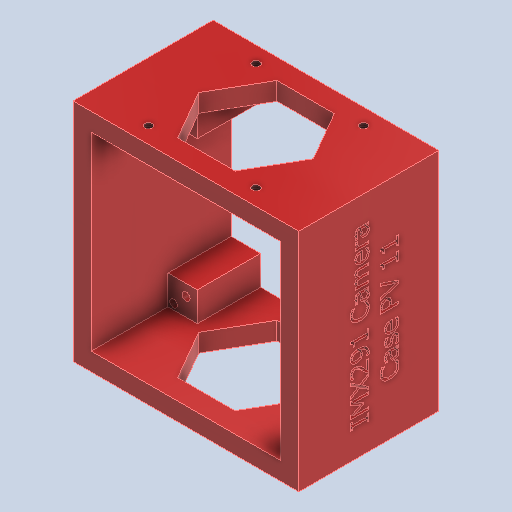
# Autodesk Inventor part: IMX291 Camera Case Base
Saved by Autodesk Inventor 2023 (Build 270158030, 158C)
## iProperties
Created: 2021-07-23
Part Number: IMX291 Camera Case Base
Material: PET Plastic
Document SubType Name: Modeling
Designer: robst
Density: 1.541 g/cm^3
Appearance: Red
Author: robst
Autodesk Inventor part; units mm, degrees
note: some values were not read from the file. Chosen so that the rebuilt part matches the saved one: direction of "Emboss2"; direction of "Hole3".
ref_plane "YZ Plane" through (0, 0, 0) normal (1, 0, 0) x (0, 1, 0)
ref_plane "XZ Plane" through (0, 0, 0) normal (0, 1, 0) x (-1, 0, 0)
ref_plane "XY Plane" through (0, 0, 0) normal (0, 0, 1) x (1, 0, 0)
sketch "Sketch8" plane through (0, 0, 0) normal (0, 0, 1) x (1, 0, 0)
  line L0 (-17, -17) -> (17, -17) construction
  line L1 (17, -17) -> (17, 17) construction
  line L2 (17, 17) -> (-17, 17) construction
  line L3 (-17, 17) -> (-17, -17) construction
  line L4 (-17, -17) -> (17, 17) construction
  line L5 (17, -17) -> (-17, 17) construction
  circle A0 centre (-17, 17) radius 0.9
  circle A1 centre (17, 17) radius 0.9
  circle A2 centre (17, -17) radius 0.9
  circle A3 centre (-17, -17) radius 0.9
  line L6 (-21, -21) -> (21, -21)
  line L7 (21, -21) -> (21, 21)
  line L8 (21, 21) -> (-21, 21)
  line L9 (-21, 21) -> (-21, -21)
  line L10 (-21, -21) -> (21, 21) construction
  line L11 (21, -21) -> (-21, 21) construction
  line L12 (-25, -25) -> (25, -25)
  line L13 (25, -25) -> (25, 25)
  line L14 (25, 25) -> (-25, 25)
  line L15 (-25, 25) -> (-25, -25)
  line L16 (-25, -25) -> (25, 25) construction
  line L17 (25, -25) -> (-25, 25) construction
  line L18 (0, 0) -> (9.8286, 0)
  line L19 (-14.5, -14.5) -> (14.5, -14.5) construction
  line L20 (14.5, -14.5) -> (14.5, 14.5) construction
  line L21 (14.5, 14.5) -> (-14.5, 14.5) construction
  line L22 (-14.5, 14.5) -> (-14.5, -14.5) construction
  line L23 (-14.5, -14.5) -> (14.5, 14.5) construction
  line L24 (14.5, -14.5) -> (-14.5, 14.5) construction
  line L25 (-21, 21) -> (-14.5, 21)
  line L26 (-14.5, 21) -> (-14.5, 14.5)
  line L27 (-14.5, 14.5) -> (-21, 14.5)
  line L28 (-21, 14.5) -> (-21, 21)
  line L29 (21, 21) -> (14.5, 21)
  line L30 (14.5, 21) -> (14.5, 14.5)
  line L31 (14.5, 14.5) -> (21, 14.5)
  line L32 (21, 14.5) -> (21, 21)
  line L33 (21, -21) -> (14.5, -21)
  line L34 (14.5, -21) -> (14.5, -14.5)
  line L35 (14.5, -14.5) -> (21, -14.5)
  line L36 (21, -14.5) -> (21, -21)
  line L37 (-21, -21) -> (-14.5, -21)
  line L38 (-14.5, -21) -> (-14.5, -14.5)
  line L39 (-14.5, -14.5) -> (-21, -14.5)
  line L40 (-21, -14.5) -> (-21, -21)
  point P0 (-25, 0)
  point P1 (-14.5, -21)
  dimension "d46" = 34
  dimension "d47" = 34
  dimension "d48" = 1.8
  dimension "d49" = 42
  dimension "d50" = 42
  dimension "d51" = 4
  dimension "d52" = 4
  dimension "d53" = 29
  dimension "d54" = 29
  dimension "d61" = 50
  dimension "d62" = 50
  constraints: 82 end point, 16 parallel, 9 midpoint, 8 horizontal, 8 perpendicular, 4 centre point, 4 coincident, 3 equal radius, 2 point on line
  measures "d46" distance of L0.start L0.end
  measures "d47" distance of L2.end L0.start
  measures "d48" diameter of A0
  measures "d49" distance of L7.end L8.end
  measures "d50" distance of L6.end L7.end
  measures "d51" distance between parallel lines of L8 L14
  measures "d52" distance from line of point (-25, 0) L9
  measures "d53" distance of L19.start L19.end
  measures "d54" distance of L20.end L19.end
  measures "d61" distance between parallel lines of L14 L12
  measures "d62" distance between parallel lines of L15 L13
extrude "Extrusion9" add sketch "Sketch8" against normal blind 14 contours L9 L39 L38 L6 | L34 L35 L7 L6 | L9 L8 L26 L27 | L31 L30 L8 L7 | L15 L14 L13 L12
sketch "Sketch9" plane through (0, 0, 0) normal (0, 0, 1) x (1, 0, 0)
  line L0 (21, 14.5) -> (21, -14.5) projected
  line L1 (-14.5, 21) -> (14.5, 21) projected
  line L2 (-21, -14.5) -> (-21, 14.5) projected
  line L3 (14.5, -21) -> (-14.5, -21) projected
  line L4 (-25, -25) -> (25, -25) projected
  line L5 (25, -25) -> (25, 25) projected
  line L6 (25, 25) -> (-25, 25) projected
  line L7 (-25, 25) -> (-25, -25) projected
  line L8 (-21, -21) -> (21, -21)
  line L9 (21, -21) -> (21, 21)
  line L10 (21, 21) -> (-21, 21)
  line L11 (-21, 21) -> (-21, -21)
  line L12 (-21, -21) -> (21, 21) construction
  line L13 (21, -21) -> (-21, 21) construction
  line L14 (-23, -23) -> (23, -23)
  line L15 (23, -23) -> (23, 23)
  line L16 (23, 23) -> (-23, 23)
  line L17 (-23, 23) -> (-23, -23)
  line L18 (-23, -23) -> (23, 23) construction
  line L19 (23, -23) -> (-23, 23) construction
  point P0 (0, 0)
  point P1 (-14.5, -21)
  constraints: 24 end point, 4 midpoint, 4 parallel, 2 perpendicular
extrude "Extrusion10" add sketch "Sketch9" along normal blind 17 contours L7 L6 L5 L4 | L17 L16 L15 L14
sketch "Sketch10" plane through (25, -25, -14) normal (1, 0, 0) x (0, 0, -1)
  line L0 (-31, 0) -> (0, 0) construction
  line L1 (-15.5, 0) -> (-15.5, 50) construction
  line L2 (0, 50) -> (-31, 50) construction
  line L3 (-15.5, 7.4068) -> (-15.5, 5.8574)
  line L4 (-15.5, 5.8574) -> (-15.9084, 5.8574)
  line L5 (-15.9084, 5.8574) -> (-15.9084, 6.3663)
  line L6 (-15.9084, 6.3663) -> (-19.0916, 6.3663)
  line L7 (-19.0916, 6.3663) -> (-19.0916, 5.8574)
  line L8 (-19.0916, 5.8574) -> (-19.5, 5.8574)
  line L9 (-19.5, 5.8574) -> (-19.5, 7.4068)
  line L10 (-19.5, 7.4068) -> (-19.0916, 7.4068)
  line L11 (-19.0916, 7.4068) -> (-19.0916, 6.8979)
  line L12 (-19.0916, 6.8979) -> (-15.9084, 6.8979)
  line L13 (-15.9084, 6.8979) -> (-15.9084, 7.4068)
  line L14 (-15.9084, 7.4068) -> (-15.5, 7.4068)
  line L15 (-15.5, 11.4943) -> (-15.5, 10.9627)
  line L16 (-15.5, 10.9627) -> (-18.9457, 10.9627)
  line L17 (-18.9457, 10.9627) -> (-16.6021, 9.919)
  line L18 (-16.6021, 9.919) -> (-16.6021, 9.5948)
  line L19 (-16.6021, 9.5948) -> (-18.9457, 8.5608)
  line L20 (-18.9457, 8.5608) -> (-15.5, 8.5608)
  line L21 (-15.5, 8.5608) -> (-15.5, 8.0648)
  line L22 (-15.5, 8.0648) -> (-19.5, 8.0648)
  line L23 (-19.5, 8.0648) -> (-19.5, 8.7909)
  line L24 (-19.5, 8.7909) -> (-17.2731, 9.7893)
  line L25 (-17.2731, 9.7893) -> (-19.5, 10.7553)
  line L26 (-19.5, 10.7553) -> (-19.5, 11.4943)
  line L27 (-19.5, 11.4943) -> (-15.5, 11.4943)
  line L28 (-15.5, 15.0697) -> (-15.5, 14.4603)
  line L29 (-15.5, 14.4603) -> (-17.0948, 13.4878)
  line L30 (-17.0948, 13.4878) -> (-15.5, 12.4959)
  line L31 (-15.5, 12.4959) -> (-15.5, 11.9222)
  line L32 (-15.5, 11.9222) -> (-17.5032, 13.1961)
  line L33 (-17.5032, 13.1961) -> (-19.5, 11.9611)
  line L34 (-19.5, 11.9611) -> (-19.5, 12.5705)
  line L35 (-19.5, 12.5705) -> (-17.9344, 13.5235)
  line L36 (-17.9344, 13.5235) -> (-19.5, 14.4959)
  line L37 (-19.5, 14.4959) -> (-19.5, 15.0697)
  line L38 (-19.5, 15.0697) -> (-17.5292, 13.8185)
  line L39 (-17.5292, 13.8185) -> (-15.5, 15.0697)
  line L40 (-15.5, 17.8509) -> (-15.5, 15.3841)
  line L41 (-15.5, 15.3841) -> (-16.0673, 15.3841)
  spline S0 degree 2 poles (-16.0673, 15.3841) (-16.3169, 15.6499) (-16.7804, 16.1232) (-17.03, 16.3501) knots 0 0 0 1 2 2 2
  spline S1 degree 2 poles (-17.03, 16.3501) (-17.5324, 16.8071) (-18.1353, 17.141) (-18.4562, 17.141) knots 0 0 0 1 2 2 2
  spline S2 degree 2 poles (-18.4562, 17.141) (-18.6248, 17.141) (-18.8776, 17.0373) (-18.9587, 16.9433) knots 0 0 0 1 2 2 2
  spline S3 degree 2 poles (-18.9587, 16.9433) (-19.0397, 16.8493) (-19.1207, 16.6029) (-19.1207, 16.4538) knots 0 0 0 1 2 2 2
  spline S4 degree 2 poles (-19.1207, 16.4538) (-19.1207, 16.3112) (-19.0494, 16.0194) (-18.9943, 15.8865) knots 0 0 0 1 2 2 2
  spline S5 degree 2 poles (-18.9943, 15.8865) (-18.9489, 15.7731) (-18.8193, 15.5624) (-18.7739, 15.4976) knots 0 0 0 1 2 2 2
  line L42 (-18.7739, 15.4976) -> (-18.7739, 15.4684)
  line L43 (-18.7739, 15.4684) -> (-19.3444, 15.4684)
  spline S6 degree 2 poles (-19.3444, 15.4684) (-19.4254, 15.6337) (-19.5843, 16.2269) (-19.5843, 16.4927) knots 0 0 0 1 2 2 2
  spline S7 degree 2 poles (-19.5843, 16.4927) (-19.5843, 17.0535) (-18.9911, 17.6856) (-18.4854, 17.6856) knots 0 0 0 1 2 2 2
  spline S8 degree 2 poles (-18.4854, 17.6856) (-18.2488, 17.6856) (-17.8533, 17.5754) (-17.6848, 17.4781) knots 0 0 0 1 2 2 2
  spline S9 degree 2 poles (-17.6848, 17.4781) (-17.5097, 17.3809) (-17.1661, 17.0989) (-17.0008, 16.9433) knots 0 0 0 1 2 2 2
  spline S10 degree 2 poles (-17.0008, 16.9433) (-16.7253, 16.6904) (-16.1353, 16.0713) (-15.9635, 15.8865) knots 0 0 0 1 2 2 2
  line L44 (-15.9635, 15.8865) -> (-15.9635, 17.8509)
  line L45 (-15.9635, 17.8509) -> (-15.5, 17.8509)
  spline S11 degree 2 poles (-18.2002, 18.2755) (-18.5081, 18.2755) (-19.0203, 18.4765) (-19.205, 18.6515) knots 0 0 0 1 2 2 2
  spline S12 degree 2 poles (-19.205, 18.6515) (-19.3833, 18.8169) (-19.581, 19.2998) (-19.581, 19.5462) knots 0 0 0 1 2 2 2
  spline S13 degree 2 poles (-19.581, 19.5462) (-19.581, 19.8217) (-19.3963, 20.269) (-19.2212, 20.4344) knots 0 0 0 1 2 2 2
  spline S14 degree 2 poles (-19.2212, 20.4344) (-19.0008, 20.6418) (-18.2877, 20.8687) (-17.7399, 20.8687) knots 0 0 0 1 2 2 2
  spline S15 degree 2 poles (-17.7399, 20.8687) (-17.2439, 20.8687) (-16.3558, 20.6451) (-16.0608, 20.4279) knots 0 0 0 1 2 2 2
  spline S16 degree 2 poles (-16.0608, 20.4279) (-15.7496, 20.1977) (-15.4222, 19.5494) (-15.4222, 19.0762) knots 0 0 0 1 2 2 2
  spline S17 degree 2 poles (-15.4222, 19.0762) (-15.4222, 18.9692) (-15.4449, 18.7261) (-15.4773, 18.6224) knots 0 0 0 1 2 2 2
  line L46 (-15.4773, 18.6224) -> (-15.9927, 18.6224)
  line L47 (-15.9927, 18.6224) -> (-15.9927, 18.6483)
  spline S18 degree 2 poles (-15.9927, 18.6483) (-15.9538, 18.7164) (-15.8857, 19.0016) (-15.8857, 19.1475) knots 0 0 0 1 2 2 2
  spline S19 degree 2 poles (-15.8857, 19.1475) (-15.8857, 19.6726) (-16.5794, 20.2723) (-17.2212, 20.3144) knots 0 0 0 1 2 2 2
  spline S20 degree 2 poles (-17.2212, 20.3144) (-17.0754, 20.1005) (-16.9425, 19.7115) (-16.9425, 19.4814) knots 0 0 0 1 2 2 2
  spline S21 degree 2 poles (-16.9425, 19.4814) (-16.9425, 19.2609) (-17.0397, 18.8947) (-17.1791, 18.7099) knots 0 0 0 1 2 2 2
  spline S22 degree 2 poles (-17.1791, 18.7099) (-17.3444, 18.4959) (-17.8468, 18.2755) (-18.2002, 18.2755) knots 0 0 0 1 2 2 2
  spline S23 degree 2 poles (-17.8598, 20.3274) (-18.265, 20.3274) (-18.7771, 20.1783) (-18.9165, 20.0454) knots 0 0 0 1 2 2 2
  spline S24 degree 2 poles (-18.9165, 20.0454) (-19.0462, 19.9287) (-19.1434, 19.6856) (-19.1434, 19.5429) knots 0 0 0 1 2 2 2
  spline S25 degree 2 poles (-19.1434, 19.5429) (-19.1434, 19.2123) (-18.6702, 18.8201) (-18.2229, 18.8201) knots 0 0 0 1 2 2 2
  spline S26 degree 2 poles (-18.2229, 18.8201) (-17.97, 18.8201) (-17.6426, 18.9498) (-17.5259, 19.0924) knots 0 0 0 1 2 2 2
  spline S27 degree 2 poles (-17.5259, 19.0924) (-17.4417, 19.1961) (-17.3865, 19.4522) (-17.3865, 19.6013) knots 0 0 0 1 2 2 2
  spline S28 degree 2 poles (-17.3865, 19.6013) (-17.3865, 19.7731) (-17.5065, 20.1686) (-17.607, 20.3177) knots 0 0 0 1 2 2 2
  spline S29 degree 2 poles (-17.607, 20.3177) (-17.6459, 20.3209) (-17.7788, 20.3274) (-17.8598, 20.3274) knots 0 0 0 1 2 2 2
  line L48 (-15.5, 23.6532) -> (-15.5, 21.7018)
  line L49 (-15.5, 21.7018) -> (-15.9084, 21.7018)
  line L50 (-15.9084, 21.7018) -> (-15.9084, 22.4279)
  line L51 (-15.9084, 22.4279) -> (-18.5891, 22.4279)
  line L52 (-18.5891, 22.4279) -> (-18.5891, 21.7018)
  line L53 (-18.5891, 21.7018) -> (-18.9554, 21.7018)
  spline S30 degree 2 poles (-18.9554, 21.7018) (-18.9554, 22.1135) (-19.1888, 22.5024) (-19.513, 22.5284) knots 0 0 0 1 2 2 2
  line L54 (-19.513, 22.5284) -> (-19.513, 22.9433)
  line L55 (-19.513, 22.9433) -> (-15.9084, 22.9433)
  line L56 (-15.9084, 22.9433) -> (-15.9084, 23.6532)
  line L57 (-15.9084, 23.6532) -> (-15.5, 23.6532)
  spline S31 degree 2 poles (-15.4287, 27.7828) (-15.4287, 27.3938) (-15.6912, 26.7358) (-15.9538, 26.4959) knots 0 0 0 1 2 2 2
  spline S32 degree 2 poles (-15.9538, 26.4959) (-16.2131, 26.2561) (-16.9911, 25.9935) (-17.4968, 25.9935) knots 0 0 0 1 2 2 2
  spline S33 degree 2 poles (-17.4968, 25.9935) (-17.9992, 25.9935) (-18.7447, 26.2496) (-19.0203, 26.4927) knots 0 0 0 1 2 2 2
  spline S34 degree 2 poles (-19.0203, 26.4927) (-19.2893, 26.7326) (-19.5713, 27.3874) (-19.5713, 27.7925) knots 0 0 0 1 2 2 2
  spline S35 degree 2 poles (-19.5713, 27.7925) (-19.5713, 27.9935) (-19.513, 28.3468) (-19.4676, 28.4959) knots 0 0 0 1 2 2 2
  spline S36 degree 2 poles (-19.4676, 28.4959) (-19.4254, 28.6256) (-19.3055, 28.8947) (-19.2342, 29.0276) knots 0 0 0 1 2 2 2
  line L58 (-19.2342, 29.0276) -> (-18.5924, 29.0276)
  line L59 (-18.5924, 29.0276) -> (-18.5924, 28.9854)
  spline S37 degree 2 poles (-18.5924, 28.9854) (-18.6572, 28.9141) (-18.8387, 28.6937) (-18.9263, 28.5348) knots 0 0 0 1 2 2 2
  spline S38 degree 2 poles (-18.9263, 28.5348) (-19.0105, 28.3825) (-19.1175, 28.0227) (-19.1175, 27.7893) knots 0 0 0 1 2 2 2
  spline S39 degree 2 poles (-19.1175, 27.7893) (-19.1175, 27.5332) (-18.9068, 27.0762) (-18.7058, 26.9044) knots 0 0 0 1 2 2 2
  spline S40 degree 2 poles (-18.7058, 26.9044) (-18.5016, 26.7358) (-17.8825, 26.5478) (-17.4968, 26.5478) knots 0 0 0 1 2 2 2
  spline S41 degree 2 poles (-17.4968, 26.5478) (-17.0851, 26.5478) (-16.4919, 26.7455) (-16.2877, 26.9173) knots 0 0 0 1 2 2 2
  spline S42 degree 2 poles (-16.2877, 26.9173) (-16.09, 27.0859) (-15.889, 27.5365) (-15.889, 27.7893) knots 0 0 0 1 2 2 2
  spline S43 degree 2 poles (-15.889, 27.7893) (-15.889, 28.0194) (-16.0024, 28.4117) (-16.0867, 28.564) knots 0 0 0 1 2 2 2
  spline S44 degree 2 poles (-16.0867, 28.564) (-16.171, 28.7099) (-16.346, 28.9271) (-16.4076, 28.9887) knots 0 0 0 1 2 2 2
  line L60 (-16.4076, 28.9887) -> (-16.4076, 29.0276)
  line L61 (-16.4076, 29.0276) -> (-15.7723, 29.0276)
  spline S45 degree 2 poles (-15.7723, 29.0276) (-15.7107, 28.8947) (-15.5972, 28.6613) (-15.5454, 28.4959) knots 0 0 0 1 2 2 2
  spline S46 degree 2 poles (-15.5454, 28.4959) (-15.487, 28.3209) (-15.4287, 28.0227) (-15.4287, 27.7828) knots 0 0 0 1 2 2 2
  spline S47 degree 2 poles (-15.8177, 31.1572) (-15.7723, 31.0956) (-15.6102, 30.8882) (-15.5616, 30.7909) knots 0 0 0 1 2 2 2
  spline S48 degree 2 poles (-15.5616, 30.7909) (-15.4903, 30.658) (-15.4157, 30.4084) (-15.4157, 30.1815) knots 0 0 0 1 2 2 2
  spline S49 degree 2 poles (-15.4157, 30.1815) (-15.4157, 29.9968) (-15.5551, 29.6629) (-15.6815, 29.5365) knots 0 0 0 1 2 2 2
  spline S50 degree 2 poles (-15.6815, 29.5365) (-15.8047, 29.4165) (-16.1677, 29.2707) (-16.3687, 29.2707) knots 0 0 0 1 2 2 2
  spline S51 degree 2 poles (-16.3687, 29.2707) (-16.6799, 29.2707) (-17.1207, 29.5332) (-17.2472, 29.8185) knots 0 0 0 1 2 2 2
  spline S52 degree 2 poles (-17.2472, 29.8185) (-17.3639, 30.0713) (-17.4514, 30.7585) (-17.4741, 31.1572) knots 0 0 0 1 2 2 2
  line L62 (-17.4741, 31.1572) -> (-17.5713, 31.1572)
  spline S53 degree 2 poles (-17.5713, 31.1572) (-17.7464, 31.1572) (-17.9635, 31.0502) (-18.0251, 30.953) knots 0 0 0 1 2 2 2
  spline S54 degree 2 poles (-18.0251, 30.953) (-18.0867, 30.8558) (-18.1256, 30.577) (-18.1256, 30.4279) knots 0 0 0 1 2 2 2
  spline S55 degree 2 poles (-18.1256, 30.4279) (-18.1256, 30.2528) (-18.0219, 29.7796) (-17.9214, 29.543) knots 0 0 0 1 2 2 2
  line L63 (-17.9214, 29.543) -> (-17.9214, 29.5138)
  line L64 (-17.9214, 29.5138) -> (-18.4368, 29.5138)
  spline S56 degree 2 poles (-18.4368, 29.5138) (-18.4757, 29.6532) (-18.5729, 30.175) (-18.5729, 30.4311) knots 0 0 0 1 2 2 2
  spline S57 degree 2 poles (-18.5729, 30.4311) (-18.5729, 30.7423) (-18.4757, 31.1669) (-18.3493, 31.3355) knots 0 0 0 1 2 2 2
  spline S58 degree 2 poles (-18.3493, 31.3355) (-18.2261, 31.5008) (-17.8339, 31.6629) (-17.5519, 31.6629) knots 0 0 0 1 2 2 2
  line L65 (-17.5519, 31.6629) -> (-15.5, 31.6629)
  line L66 (-15.5, 31.6629) -> (-15.5, 31.1572)
  line L67 (-15.5, 31.1572) -> (-15.8177, 31.1572)
  line L68 (-16.2391, 31.1572) -> (-17.0721, 31.1572)
  spline S59 degree 2 poles (-17.0721, 31.1572) (-17.0559, 30.9757) (-17.0008, 30.4279) (-16.9489, 30.2561) knots 0 0 0 1 2 2 2
  spline S60 degree 2 poles (-16.9489, 30.2561) (-16.8874, 30.0551) (-16.6313, 29.7925) (-16.4044, 29.7925) knots 0 0 0 1 2 2 2
  spline S61 degree 2 poles (-16.4044, 29.7925) (-16.1451, 29.7925) (-15.8825, 30.0843) (-15.8825, 30.363) knots 0 0 0 1 2 2 2
  spline S62 degree 2 poles (-15.8825, 30.363) (-15.8825, 30.5997) (-16.0867, 30.9887) (-16.2391, 31.1572) knots 0 0 0 1 2 2 2
  line L69 (-15.5, 35.7763) -> (-17.2374, 35.7763)
  spline S63 degree 2 poles (-17.2374, 35.7763) (-17.4449, 35.7763) (-17.7982, 35.7439) (-17.8955, 35.6921) knots 0 0 0 1 2 2 2
  spline S64 degree 2 poles (-17.8955, 35.6921) (-18.0024, 35.6402) (-18.1062, 35.4425) (-18.1062, 35.2707) knots 0 0 0 1 2 2 2
  spline S65 degree 2 poles (-18.1062, 35.2707) (-18.1062, 35.1151) (-17.9149, 34.7585) (-17.7334, 34.5705) knots 0 0 0 1 2 2 2
  spline S66 degree 2 poles (-17.7334, 34.5705) (-17.688, 34.5737) (-17.5616, 34.5802) (-17.4773, 34.5802) knots 0 0 0 1 2 2 2
  line L70 (-17.4773, 34.5802) -> (-15.5, 34.5802)
  line L71 (-15.5, 34.5802) -> (-15.5, 34.0746)
  line L72 (-15.5, 34.0746) -> (-17.2374, 34.0746)
  spline S67 degree 2 poles (-17.2374, 34.0746) (-17.4449, 34.0746) (-17.7982, 34.0421) (-17.8955, 33.9903) knots 0 0 0 1 2 2 2
  spline S68 degree 2 poles (-17.8955, 33.9903) (-18.0024, 33.9384) (-18.1062, 33.7407) (-18.1062, 33.5689) knots 0 0 0 1 2 2 2
  spline S69 degree 2 poles (-18.1062, 33.5689) (-18.1062, 33.4068) (-17.9019, 33.047) (-17.7431, 32.8784) knots 0 0 0 1 2 2 2
  line L73 (-17.7431, 32.8784) -> (-15.5, 32.8784)
  line L74 (-15.5, 32.8784) -> (-15.5, 32.3728)
  line L75 (-15.5, 32.3728) -> (-18.5016, 32.3728)
  line L76 (-18.5016, 32.3728) -> (-18.5016, 32.8784)
  line L77 (-18.5016, 32.8784) -> (-18.171, 32.8784)
  spline S70 degree 2 poles (-18.171, 32.8784) (-18.3687, 33.0762) (-18.5859, 33.4652) (-18.5859, 33.6985) knots 0 0 0 1 2 2 2
  spline S71 degree 2 poles (-18.5859, 33.6985) (-18.5859, 33.9643) (-18.3428, 34.376) (-18.0673, 34.483) knots 0 0 0 1 2 2 2
  spline S72 degree 2 poles (-18.0673, 34.483) (-18.3233, 34.7131) (-18.5859, 35.1475) (-18.5859, 35.4003) knots 0 0 0 1 2 2 2
  spline S73 degree 2 poles (-18.5859, 35.4003) (-18.5859, 35.5948) (-18.466, 35.9125) (-18.3298, 36.0292) knots 0 0 0 1 2 2 2
  spline S74 degree 2 poles (-18.3298, 36.0292) (-18.1937, 36.1491) (-17.7853, 36.282) (-17.4773, 36.282) knots 0 0 0 1 2 2 2
  line L78 (-17.4773, 36.282) -> (-15.5, 36.282)
  line L79 (-15.5, 36.282) -> (-15.5, 35.7763)
  spline S75 degree 2 poles (-15.4319, 38.295) (-15.4319, 37.5754) (-16.2391, 36.7844) (-16.9846, 36.7844) knots 0 0 0 1 2 2 2
  spline S76 degree 2 poles (-16.9846, 36.7844) (-17.7172, 36.7844) (-18.5859, 37.5527) (-18.5859, 38.1718) knots 0 0 0 1 2 2 2
  spline S77 degree 2 poles (-18.5859, 38.1718) (-18.5859, 38.4506) (-18.4238, 38.8817) (-18.252, 39.0405) knots 0 0 0 1 2 2 2
  spline S78 degree 2 poles (-18.252, 39.0405) (-18.0802, 39.2026) (-17.5843, 39.3744) (-17.2245, 39.3744) knots 0 0 0 1 2 2 2
  line L80 (-17.2245, 39.3744) -> (-16.9489, 39.3744)
  line L81 (-16.9489, 39.3744) -> (-16.9489, 37.2966)
  spline S79 degree 2 poles (-16.9489, 37.2966) (-16.4271, 37.2966) (-15.8728, 37.8217) (-15.8728, 38.2885) knots 0 0 0 1 2 2 2
  spline S80 degree 2 poles (-15.8728, 38.2885) (-15.8728, 38.4538) (-15.9473, 38.7747) (-16.0057, 38.9044) knots 0 0 0 1 2 2 2
  spline S81 degree 2 poles (-16.0057, 38.9044) (-16.0705, 39.0405) (-16.184, 39.2285) (-16.2358, 39.2901) knots 0 0 0 1 2 2 2
  line L82 (-16.2358, 39.2901) -> (-16.2358, 39.3193)
  line L83 (-16.2358, 39.3193) -> (-15.6848, 39.3193)
  spline S82 degree 2 poles (-15.6848, 39.3193) (-15.6491, 39.2318) (-15.5454, 38.966) (-15.5162, 38.8622) knots 0 0 0 1 2 2 2
  spline S83 degree 2 poles (-15.5162, 38.8622) (-15.4741, 38.7164) (-15.4319, 38.4765) (-15.4319, 38.295) knots 0 0 0 1 2 2 2
  spline S84 degree 2 poles (-17.3347, 38.8817) (-17.5389, 38.8752) (-17.8371, 38.7909) (-17.9376, 38.7099) knots 0 0 0 1 2 2 2
  spline S85 degree 2 poles (-17.9376, 38.7099) (-18.0511, 38.6224) (-18.171, 38.3468) (-18.171, 38.1426) knots 0 0 0 1 2 2 2
  spline S86 degree 2 poles (-18.171, 38.1426) (-18.171, 37.9417) (-18.0511, 37.6596) (-17.9344, 37.543) knots 0 0 0 1 2 2 2
  spline S87 degree 2 poles (-17.9344, 37.543) (-17.8144, 37.4295) (-17.5259, 37.3128) (-17.3347, 37.2966) knots 0 0 0 1 2 2 2
  line L84 (-17.3347, 37.2966) -> (-17.3347, 38.8817)
  line L85 (-17.9603, 41.4781) -> (-17.9603, 41.4522)
  spline S88 degree 2 poles (-17.9603, 41.4522) (-17.9765, 41.3938) (-17.983, 41.2674) (-17.983, 41.1799) knots 0 0 0 1 2 2 2
  spline S89 degree 2 poles (-17.983, 41.1799) (-17.983, 40.9757) (-17.8047, 40.5737) (-17.6297, 40.3922) knots 0 0 0 1 2 2 2
  line L86 (-17.6297, 40.3922) -> (-15.5, 40.3922)
  line L87 (-15.5, 40.3922) -> (-15.5, 39.8865)
  line L88 (-15.5, 39.8865) -> (-18.5016, 39.8865)
  line L89 (-18.5016, 39.8865) -> (-18.5016, 40.3922)
  line L90 (-18.5016, 40.3922) -> (-18.0543, 40.3922)
  spline S90 degree 2 poles (-18.0543, 40.3922) (-18.3006, 40.6677) (-18.5016, 41.0794) (-18.5016, 41.2739) knots 0 0 0 1 2 2 2
  spline S91 degree 2 poles (-18.5016, 41.2739) (-18.5016, 41.3517) (-18.4951, 41.4295) (-18.4854, 41.4781) knots 0 0 0 1 2 2 2
  line L91 (-18.4854, 41.4781) -> (-17.9603, 41.4781)
  spline S92 degree 2 poles (-15.8177, 43.543) (-15.7723, 43.4814) (-15.6102, 43.2739) (-15.5616, 43.1767) knots 0 0 0 1 2 2 2
  spline S93 degree 2 poles (-15.5616, 43.1767) (-15.4903, 43.0438) (-15.4157, 42.7942) (-15.4157, 42.5673) knots 0 0 0 1 2 2 2
  spline S94 degree 2 poles (-15.4157, 42.5673) (-15.4157, 42.3825) (-15.5551, 42.0486) (-15.6815, 41.9222) knots 0 0 0 1 2 2 2
  spline S95 degree 2 poles (-15.6815, 41.9222) (-15.8047, 41.8023) (-16.1677, 41.6564) (-16.3687, 41.6564) knots 0 0 0 1 2 2 2
  spline S96 degree 2 poles (-16.3687, 41.6564) (-16.6799, 41.6564) (-17.1207, 41.919) (-17.2472, 42.2042) knots 0 0 0 1 2 2 2
  spline S97 degree 2 poles (-17.2472, 42.2042) (-17.3639, 42.4571) (-17.4514, 43.1442) (-17.4741, 43.543) knots 0 0 0 1 2 2 2
  line L92 (-17.4741, 43.543) -> (-17.5713, 43.543)
  spline S98 degree 2 poles (-17.5713, 43.543) (-17.7464, 43.543) (-17.9635, 43.436) (-18.0251, 43.3387) knots 0 0 0 1 2 2 2
  spline S99 degree 2 poles (-18.0251, 43.3387) (-18.0867, 43.2415) (-18.1256, 42.9627) (-18.1256, 42.8136) knots 0 0 0 1 2 2 2
  spline S100 degree 2 poles (-18.1256, 42.8136) (-18.1256, 42.6386) (-18.0219, 42.1653) (-17.9214, 41.9287) knots 0 0 0 1 2 2 2
  line L93 (-17.9214, 41.9287) -> (-17.9214, 41.8995)
  line L94 (-17.9214, 41.8995) -> (-18.4368, 41.8995)
  spline S101 degree 2 poles (-18.4368, 41.8995) (-18.4757, 42.0389) (-18.5729, 42.5608) (-18.5729, 42.8169) knots 0 0 0 1 2 2 2
  spline S102 degree 2 poles (-18.5729, 42.8169) (-18.5729, 43.128) (-18.4757, 43.5527) (-18.3493, 43.7212) knots 0 0 0 1 2 2 2
  spline S103 degree 2 poles (-18.3493, 43.7212) (-18.2261, 43.8865) (-17.8339, 44.0486) (-17.5519, 44.0486) knots 0 0 0 1 2 2 2
  line L95 (-17.5519, 44.0486) -> (-15.5, 44.0486)
  line L96 (-15.5, 44.0486) -> (-15.5, 43.543)
  line L97 (-15.5, 43.543) -> (-15.8177, 43.543)
  line L98 (-16.2391, 43.543) -> (-17.0721, 43.543)
  spline S104 degree 2 poles (-17.0721, 43.543) (-17.0559, 43.3614) (-17.0008, 42.8136) (-16.9489, 42.6418) knots 0 0 0 1 2 2 2
  spline S105 degree 2 poles (-16.9489, 42.6418) (-16.8874, 42.4408) (-16.6313, 42.1783) (-16.4044, 42.1783) knots 0 0 0 1 2 2 2
  spline S106 degree 2 poles (-16.4044, 42.1783) (-16.1451, 42.1783) (-15.8825, 42.47) (-15.8825, 42.7488) knots 0 0 0 1 2 2 2
  spline S107 degree 2 poles (-15.8825, 42.7488) (-15.8825, 42.9854) (-16.0867, 43.3744) (-16.2391, 43.543) knots 0 0 0 1 2 2 2
  spline S108 degree 2 poles (-8.8362, 13.3193) (-8.8362, 12.9303) (-9.0988, 12.2723) (-9.3613, 12.0324) knots 0 0 0 1 2 2 2
  spline S109 degree 2 poles (-9.3613, 12.0324) (-9.6207, 11.7925) (-10.3986, 11.53) (-10.9043, 11.53) knots 0 0 0 1 2 2 2
  spline S110 degree 2 poles (-10.9043, 11.53) (-11.4067, 11.53) (-12.1523, 11.7861) (-12.4278, 12.0292) knots 0 0 0 1 2 2 2
  spline S111 degree 2 poles (-12.4278, 12.0292) (-12.6968, 12.269) (-12.9788, 12.9238) (-12.9788, 13.329) knots 0 0 0 1 2 2 2
  spline S112 degree 2 poles (-12.9788, 13.329) (-12.9788, 13.53) (-12.9205, 13.8833) (-12.8751, 14.0324) knots 0 0 0 1 2 2 2
  spline S113 degree 2 poles (-12.8751, 14.0324) (-12.833, 14.1621) (-12.713, 14.4311) (-12.6417, 14.564) knots 0 0 0 1 2 2 2
  line L99 (-12.6417, 14.564) -> (-11.9999, 14.564)
  line L100 (-11.9999, 14.564) -> (-11.9999, 14.5219)
  spline S114 degree 2 poles (-11.9999, 14.5219) (-12.0647, 14.4506) (-12.2463, 14.2301) (-12.3338, 14.0713) knots 0 0 0 1 2 2 2
  spline S115 degree 2 poles (-12.3338, 14.0713) (-12.4181, 13.919) (-12.525, 13.5592) (-12.525, 13.3258) knots 0 0 0 1 2 2 2
  spline S116 degree 2 poles (-12.525, 13.3258) (-12.525, 13.0697) (-12.3143, 12.6126) (-12.1134, 12.4408) knots 0 0 0 1 2 2 2
  spline S117 degree 2 poles (-12.1134, 12.4408) (-11.9091, 12.2723) (-11.29, 12.0843) (-10.9043, 12.0843) knots 0 0 0 1 2 2 2
  spline S118 degree 2 poles (-10.9043, 12.0843) (-10.4926, 12.0843) (-9.8994, 12.282) (-9.6952, 12.4538) knots 0 0 0 1 2 2 2
  spline S119 degree 2 poles (-9.6952, 12.4538) (-9.4975, 12.6224) (-9.2965, 13.0729) (-9.2965, 13.3258) knots 0 0 0 1 2 2 2
  spline S120 degree 2 poles (-9.2965, 13.3258) (-9.2965, 13.5559) (-9.41, 13.9481) (-9.4942, 14.1005) knots 0 0 0 1 2 2 2
  spline S121 degree 2 poles (-9.4942, 14.1005) (-9.5785, 14.2464) (-9.7536, 14.4635) (-9.8151, 14.5251) knots 0 0 0 1 2 2 2
  line L101 (-9.8151, 14.5251) -> (-9.8151, 14.564)
  line L102 (-9.8151, 14.564) -> (-9.1798, 14.564)
  spline S122 degree 2 poles (-9.1798, 14.564) (-9.1182, 14.4311) (-9.0048, 14.1977) (-8.9529, 14.0324) knots 0 0 0 1 2 2 2
  spline S123 degree 2 poles (-8.9529, 14.0324) (-8.8946, 13.8574) (-8.8362, 13.5592) (-8.8362, 13.3193) knots 0 0 0 1 2 2 2
  spline S124 degree 2 poles (-9.2252, 16.6937) (-9.1798, 16.6321) (-9.0177, 16.4246) (-8.9691, 16.3274) knots 0 0 0 1 2 2 2
  spline S125 degree 2 poles (-8.9691, 16.3274) (-8.8978, 16.1945) (-8.8233, 15.9449) (-8.8233, 15.718) knots 0 0 0 1 2 2 2
  spline S126 degree 2 poles (-8.8233, 15.718) (-8.8233, 15.5332) (-8.9626, 15.1994) (-9.0891, 15.0729) knots 0 0 0 1 2 2 2
  spline S127 degree 2 poles (-9.0891, 15.0729) (-9.2122, 14.953) (-9.5753, 14.8071) (-9.7762, 14.8071) knots 0 0 0 1 2 2 2
  spline S128 degree 2 poles (-9.7762, 14.8071) (-10.0874, 14.8071) (-10.5283, 15.0697) (-10.6547, 15.3549) knots 0 0 0 1 2 2 2
  spline S129 degree 2 poles (-10.6547, 15.3549) (-10.7714, 15.6078) (-10.8589, 16.295) (-10.8816, 16.6937) knots 0 0 0 1 2 2 2
  line L103 (-10.8816, 16.6937) -> (-10.9788, 16.6937)
  spline S130 degree 2 poles (-10.9788, 16.6937) (-11.1539, 16.6937) (-11.3711, 16.5867) (-11.4327, 16.4895) knots 0 0 0 1 2 2 2
  spline S131 degree 2 poles (-11.4327, 16.4895) (-11.4942, 16.3922) (-11.5331, 16.1135) (-11.5331, 15.9643) knots 0 0 0 1 2 2 2
  spline S132 degree 2 poles (-11.5331, 15.9643) (-11.5331, 15.7893) (-11.4294, 15.316) (-11.3289, 15.0794) knots 0 0 0 1 2 2 2
  line L104 (-11.3289, 15.0794) -> (-11.3289, 15.0502)
  line L105 (-11.3289, 15.0502) -> (-11.8443, 15.0502)
  spline S133 degree 2 poles (-11.8443, 15.0502) (-11.8832, 15.1896) (-11.9805, 15.7115) (-11.9805, 15.9676) knots 0 0 0 1 2 2 2
  spline S134 degree 2 poles (-11.9805, 15.9676) (-11.9805, 16.2788) (-11.8832, 16.7034) (-11.7568, 16.872) knots 0 0 0 1 2 2 2
  spline S135 degree 2 poles (-11.7568, 16.872) (-11.6336, 17.0373) (-11.2414, 17.1994) (-10.9594, 17.1994) knots 0 0 0 1 2 2 2
  line L106 (-10.9594, 17.1994) -> (-8.9075, 17.1994)
  line L107 (-8.9075, 17.1994) -> (-8.9075, 16.6937)
  line L108 (-8.9075, 16.6937) -> (-9.2252, 16.6937)
  line L109 (-9.6466, 16.6937) -> (-10.4797, 16.6937)
  spline S136 degree 2 poles (-10.4797, 16.6937) (-10.4634, 16.5122) (-10.4083, 15.9643) (-10.3565, 15.7925) knots 0 0 0 1 2 2 2
  spline S137 degree 2 poles (-10.3565, 15.7925) (-10.2949, 15.5916) (-10.0388, 15.329) (-9.8119, 15.329) knots 0 0 0 1 2 2 2
  spline S138 degree 2 poles (-9.8119, 15.329) (-9.5526, 15.329) (-9.29, 15.6207) (-9.29, 15.8995) knots 0 0 0 1 2 2 2
  spline S139 degree 2 poles (-9.29, 15.8995) (-9.29, 16.1361) (-9.4942, 16.5251) (-9.6466, 16.6937) knots 0 0 0 1 2 2 2
  spline S140 degree 2 poles (-8.8362, 18.7196) (-8.8362, 18.4182) (-8.9983, 17.8963) (-9.0891, 17.7245) knots 0 0 0 1 2 2 2
  line L110 (-9.0891, 17.7245) -> (-9.6563, 17.7245)
  line L111 (-9.6563, 17.7245) -> (-9.6563, 17.7504)
  spline S141 degree 2 poles (-9.6563, 17.7504) (-9.6044, 17.8152) (-9.4813, 17.9903) (-9.4132, 18.1361) knots 0 0 0 1 2 2 2
  spline S142 degree 2 poles (-9.4132, 18.1361) (-9.3516, 18.2626) (-9.2609, 18.5737) (-9.2609, 18.7391) knots 0 0 0 1 2 2 2
  spline S143 degree 2 poles (-9.2609, 18.7391) (-9.2609, 18.859) (-9.316, 19.1345) (-9.3613, 19.1994) knots 0 0 0 1 2 2 2
  spline S144 degree 2 poles (-9.3613, 19.1994) (-9.4229, 19.2934) (-9.5623, 19.3776) (-9.7049, 19.3776) knots 0 0 0 1 2 2 2
  spline S145 degree 2 poles (-9.7049, 19.3776) (-9.8832, 19.3776) (-10.068, 19.1831) (-10.1296, 18.9335) knots 0 0 0 1 2 2 2
  spline S146 degree 2 poles (-10.1296, 18.9335) (-10.1523, 18.8363) (-10.2171, 18.5251) (-10.2527, 18.3922) knots 0 0 0 1 2 2 2
  spline S147 degree 2 poles (-10.2527, 18.3922) (-10.3532, 18.0486) (-10.7681, 17.7374) (-11.0631, 17.7374) knots 0 0 0 1 2 2 2
  spline S148 degree 2 poles (-11.0631, 17.7374) (-11.4715, 17.7374) (-11.9805, 18.3501) (-11.9805, 18.8558) knots 0 0 0 1 2 2 2
  spline S149 degree 2 poles (-11.9805, 18.8558) (-11.9805, 19.1053) (-11.8573, 19.611) (-11.7633, 19.7828) knots 0 0 0 1 2 2 2
  line L112 (-11.7633, 19.7828) -> (-11.222, 19.7828)
  line L113 (-11.222, 19.7828) -> (-11.222, 19.7569)
  spline S150 degree 2 poles (-11.222, 19.7569) (-11.3775, 19.5624) (-11.5558, 19.0891) (-11.5558, 18.846) knots 0 0 0 1 2 2 2
  spline S151 degree 2 poles (-11.5558, 18.846) (-11.5558, 18.5964) (-11.3451, 18.2528) (-11.1344, 18.2528) knots 0 0 0 1 2 2 2
  spline S152 degree 2 poles (-11.1344, 18.2528) (-10.9432, 18.2528) (-10.7584, 18.457) (-10.7001, 18.684) knots 0 0 0 1 2 2 2
  spline S153 degree 2 poles (-10.7001, 18.684) (-10.6709, 18.7942) (-10.6126, 19.0729) (-10.5769, 19.2253) knots 0 0 0 1 2 2 2
  spline S154 degree 2 poles (-10.5769, 19.2253) (-10.4926, 19.5559) (-10.1069, 19.893) (-9.773, 19.893) knots 0 0 0 1 2 2 2
  spline S155 degree 2 poles (-9.773, 19.893) (-9.5785, 19.893) (-9.2349, 19.7407) (-9.1085, 19.5916) knots 0 0 0 1 2 2 2
  spline S156 degree 2 poles (-9.1085, 19.5916) (-8.9756, 19.4327) (-8.8362, 19.0276) (-8.8362, 18.7196) knots 0 0 0 1 2 2 2
  spline S157 degree 2 poles (-8.8395, 21.6661) (-8.8395, 20.9465) (-9.6466, 20.1556) (-10.3921, 20.1556) knots 0 0 0 1 2 2 2
  spline S158 degree 2 poles (-10.3921, 20.1556) (-11.1247, 20.1556) (-11.9934, 20.9238) (-11.9934, 21.5429) knots 0 0 0 1 2 2 2
  spline S159 degree 2 poles (-11.9934, 21.5429) (-11.9934, 21.8217) (-11.8314, 22.2528) (-11.6596, 22.4117) knots 0 0 0 1 2 2 2
  spline S160 degree 2 poles (-11.6596, 22.4117) (-11.4878, 22.5737) (-10.9918, 22.7455) (-10.632, 22.7455) knots 0 0 0 1 2 2 2
  line L114 (-10.632, 22.7455) -> (-10.3565, 22.7455)
  line L115 (-10.3565, 22.7455) -> (-10.3565, 20.6677)
  spline S161 degree 2 poles (-10.3565, 20.6677) (-9.8346, 20.6677) (-9.2803, 21.1929) (-9.2803, 21.6596) knots 0 0 0 1 2 2 2
  spline S162 degree 2 poles (-9.2803, 21.6596) (-9.2803, 21.825) (-9.3549, 22.1459) (-9.4132, 22.2755) knots 0 0 0 1 2 2 2
  spline S163 degree 2 poles (-9.4132, 22.2755) (-9.478, 22.4117) (-9.5915, 22.5997) (-9.6433, 22.6613) knots 0 0 0 1 2 2 2
  line L116 (-9.6433, 22.6613) -> (-9.6433, 22.6904)
  line L117 (-9.6433, 22.6904) -> (-9.0923, 22.6904)
  spline S164 degree 2 poles (-9.0923, 22.6904) (-9.0566, 22.6029) (-8.9529, 22.3371) (-8.9237, 22.2334) knots 0 0 0 1 2 2 2
  spline S165 degree 2 poles (-8.9237, 22.2334) (-8.8816, 22.0875) (-8.8395, 21.8476) (-8.8395, 21.6661) knots 0 0 0 1 2 2 2
  spline S166 degree 2 poles (-10.7422, 22.2528) (-10.9464, 22.2464) (-11.2446, 22.1621) (-11.3451, 22.081) knots 0 0 0 1 2 2 2
  spline S167 degree 2 poles (-11.3451, 22.081) (-11.4586, 21.9935) (-11.5785, 21.718) (-11.5785, 21.5138) knots 0 0 0 1 2 2 2
  spline S168 degree 2 poles (-11.5785, 21.5138) (-11.5785, 21.3128) (-11.4586, 21.0308) (-11.3419, 20.9141) knots 0 0 0 1 2 2 2
  spline S169 degree 2 poles (-11.3419, 20.9141) (-11.222, 20.8006) (-10.9335, 20.684) (-10.7422, 20.6677) knots 0 0 0 1 2 2 2
  line L118 (-10.7422, 20.6677) -> (-10.7422, 22.2528)
  spline S170 degree 2 poles (-11.7017, 27.5429) (-11.4424, 27.5429) (-10.9756, 27.3582) (-10.8135, 27.1929) knots 0 0 0 1 2 2 2
  spline S171 degree 2 poles (-10.8135, 27.1929) (-10.6093, 26.9854) (-10.3986, 26.4246) (-10.3986, 25.9968) knots 0 0 0 1 2 2 2
  line L119 (-10.3986, 25.9968) -> (-10.3986, 25.5462)
  line L120 (-10.3986, 25.5462) -> (-8.9075, 25.5462)
  line L121 (-8.9075, 25.5462) -> (-8.9075, 25.0146)
  line L122 (-8.9075, 25.0146) -> (-12.9075, 25.0146)
  line L123 (-12.9075, 25.0146) -> (-12.9075, 26.0194)
  spline S172 degree 2 poles (-12.9075, 26.0194) (-12.9075, 26.376) (-12.7908, 26.8752) (-12.6579, 27.0665) knots 0 0 0 1 2 2 2
  spline S173 degree 2 poles (-12.6579, 27.0665) (-12.5056, 27.2901) (-12.0356, 27.5429) (-11.7017, 27.5429) knots 0 0 0 1 2 2 2
  spline S174 degree 2 poles (-11.6855, 26.9887) (-11.8929, 26.9887) (-12.1976, 26.846) (-12.2949, 26.7002) knots 0 0 0 1 2 2 2
  spline S175 degree 2 poles (-12.2949, 26.7002) (-12.3792, 26.5737) (-12.4472, 26.2366) (-12.4472, 25.987) knots 0 0 0 1 2 2 2
  line L124 (-12.4472, 25.987) -> (-12.4472, 25.5462)
  line L125 (-12.4472, 25.5462) -> (-10.8524, 25.5462)
  line L126 (-10.8524, 25.5462) -> (-10.8524, 25.9092)
  spline S176 degree 2 poles (-10.8524, 25.9092) (-10.8524, 26.2334) (-10.9562, 26.6321) (-11.0923, 26.7618) knots 0 0 0 1 2 2 2
  spline S177 degree 2 poles (-11.0923, 26.7618) (-11.2122, 26.8817) (-11.4942, 26.9887) (-11.6855, 26.9887) knots 0 0 0 1 2 2 2
  line L127 (-12.9075, 30.9498) -> (-8.9075, 29.5721)
  line L128 (-8.9075, 29.5721) -> (-8.9075, 28.9984)
  line L129 (-8.9075, 28.9984) -> (-12.9075, 27.6207)
  line L130 (-12.9075, 27.6207) -> (-12.9075, 28.1912)
  line L131 (-12.9075, 28.1912) -> (-9.585, 29.2998)
  line L132 (-9.585, 29.2998) -> (-12.9075, 30.4084)
  line L133 (-12.9075, 30.4084) -> (-12.9075, 30.9498)
  line L134 (-8.9075, 35.248) -> (-8.9075, 33.2966)
  line L135 (-8.9075, 33.2966) -> (-9.316, 33.2966)
  line L136 (-9.316, 33.2966) -> (-9.316, 34.0227)
  line L137 (-9.316, 34.0227) -> (-11.9967, 34.0227)
  line L138 (-11.9967, 34.0227) -> (-11.9967, 33.2966)
  line L139 (-11.9967, 33.2966) -> (-12.363, 33.2966)
  spline S178 degree 2 poles (-12.363, 33.2966) (-12.363, 33.7083) (-12.5963, 34.0972) (-12.9205, 34.1232) knots 0 0 0 1 2 2 2
  line L140 (-12.9205, 34.1232) -> (-12.9205, 34.5381)
  line L141 (-12.9205, 34.5381) -> (-9.316, 34.5381)
  line L142 (-9.316, 34.5381) -> (-9.316, 35.248)
  line L143 (-9.316, 35.248) -> (-8.9075, 35.248)
  line L144 (-8.9075, 38.2496) -> (-8.9075, 36.2982)
  line L145 (-8.9075, 36.2982) -> (-9.316, 36.2982)
  line L146 (-9.316, 36.2982) -> (-9.316, 37.0243)
  line L147 (-9.316, 37.0243) -> (-11.9967, 37.0243)
  line L148 (-11.9967, 37.0243) -> (-11.9967, 36.2982)
  line L149 (-11.9967, 36.2982) -> (-12.363, 36.2982)
  spline S179 degree 2 poles (-12.363, 36.2982) (-12.363, 36.7099) (-12.5963, 37.0989) (-12.9205, 37.1248) knots 0 0 0 1 2 2 2
  line L150 (-12.9205, 37.1248) -> (-12.9205, 37.5397)
  line L151 (-12.9205, 37.5397) -> (-9.316, 37.5397)
  line L152 (-9.316, 37.5397) -> (-9.316, 38.2496)
  line L153 (-9.316, 38.2496) -> (-8.9075, 38.2496)
  point P0 (-14, 25)
  constraints: 2 end point, 2 midpoint, 1 vertical
emboss "Emboss2" sketch "Sketch10" operation cut depth 1 direction (-1, 0, 0)
sketch "Sketch11" plane through (0, 0, -14) normal (0, 0, -1) x (-1, 0, 0)
  line L0 (25, -25) -> (25, 25) projected
  line L1 (-25, -25) -> (25, -25) projected
  line L2 (-25, 25) -> (-25, -25) projected
  line L3 (25, 25) -> (-25, 25) projected
  line L4 (-19.75, 19.75) -> (-19.75, -19.75) construction
  line L5 (-19.75, -19.75) -> (19.75, -19.75) construction
  line L6 (19.75, -19.75) -> (19.75, 19.75) construction
  line L7 (19.75, 19.75) -> (-19.75, 19.75) construction
  line L8 (-19.75, 19.75) -> (19.75, -19.75) construction
  line L9 (-19.75, -19.75) -> (19.75, 19.75) construction
  point P0 (0, 0)
  dimension "d74" = 39.5
  dimension "d75" = 39.5
  constraints: 12 end point, 4 coincident, 2 midpoint, 2 parallel, 1 perpendicular, 1 vertical
  measures "d74" distance of L5.end L6.end
  measures "d75" distance of L6.end L4.start
hole "Hole1" at (-19.75, 19.75, -14) at (-19.75, -19.75, -14) at (19.75, -19.75, -14) at (19.75, 19.75, -14) direction (0, 0, 1) diameter 1.6942 end through all thread size "2-56 UNC" class "3B" standard "ANSI Unified Screw Threads"
sketch "Sketch14" plane through (-25, 25, -14) normal (0, 1, 0) x (1, 0, 0)
  line L0 (50, -31) -> (0, -31) projected
  line L1 (50, 0) -> (50, -31) projected
  line L2 (0, 0) -> (50, 0) projected
  line L3 (0, 0) -> (0, -31) projected
  line L4 (50, 0) -> (0, 0) construction
  line L5 (0, 0) -> (0, -31) construction
  line L6 (50, 0) -> (0, -31) construction
  line L7 (50, -31) -> (0, 0) construction
  line L8 (37.7017, -15.5) -> (31.3509, -26.5)
  line L9 (31.3509, -26.5) -> (18.6491, -26.5)
  line L10 (18.6491, -26.5) -> (12.2983, -15.5)
  line L11 (12.2983, -15.5) -> (18.6491, -4.5)
  line L12 (18.6491, -4.5) -> (31.3509, -4.5)
  line L13 (31.3509, -4.5) -> (37.7017, -15.5)
  point P0 (25, -14)
  point P1 (25, -15.5)
  point P2 (25, -15.5)
  dimension "d101" = 22
  constraints: 16 end point, 1 coincident, 1 horizontal, 1 midpoint, 13 other
  measures "d101" distance between parallel lines of L9 L12
sketch "Sketch15" plane through (-25, 25, -14) normal (0, 1, 0) x (1, 0, 0)
  line L0 (0, 0) -> (50, 0) projected
  line L1 (50, 0) -> (50, -31) projected
  line L2 (50, -31) -> (0, -31) projected
  line L3 (0, 0) -> (0, -31) projected
  line L4 (0, 0) -> (50, -31) construction
  line L5 (50, 0) -> (0, -31) construction
  line L6 (13.1, -27.4) -> (36.9, -27.4) construction
  line L7 (36.9, -27.4) -> (36.9, -3.6) construction
  line L8 (36.9, -3.6) -> (13.1, -3.6) construction
  line L9 (13.1, -3.6) -> (13.1, -27.4) construction
  line L10 (13.1, -27.4) -> (36.9, -3.6) construction
  line L11 (36.9, -27.4) -> (13.1, -3.6) construction
  point P0 (25, -14)
  point P1 (25, -15.5)
  dimension "d93" = 23.8
  constraints: 16 end point, 4 coincident, 3 midpoint, 2 parallel, 2 perpendicular, 1 horizontal
  measures "d93" distance of L8.end L6.start
hole "Hole3" at (-11.9, 25, -10.4) at (11.9, 25, -10.4) at (11.9, 25, 13.4) at (-11.9, 25, 13.4) direction (0, -1, 0) diameter 1.6942 depth 4 thread size "2-56 UNC" class "2B" standard "ANSI Unified Screw Threads"
extrude "Extrusion13" cut sketch "Sketch14" against normal through all contours L8 L9 L10 L11 L12 L13
equation "\"d46\" = screwSpacing"
equation "\"d47\" = screwSpacing"
equation "\"d48\" = holeDiameter"
equation "\"d49\" = interiorWidth"
equation "\"d50\" = interiorWidth"
equation "\"d51\" = sideWallThickness"
equation "\"d52\" = sideWallThickness"
equation "\"d101\" = hexCoolingHole"
equation "\"screwSpacing\" = 34"
equation "\"interiorWidth\" = 42"
equation "\"bottomWallThickness\" = 2"
equation "\"holeDiameter\" = 1.8"
equation "\"sideWallThickness\" = 4"
equation "\"hexCoolingHole\" = 22"
body "Solid4"
body "Solid5"
